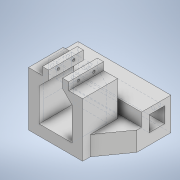
# Autodesk Inventor part: Motorhalterig
Saved by Autodesk Inventor 2021 (Build 250183000, 183)
## iProperties
Created: 2024-01-31
Part Number: Motorhalterig
Material: Generic
Document SubType Name: Modeling
Designer: Lukas
Density: 1 g/cm^3
Appearance: Default
Author: Lukas
Autodesk Inventor part; units mm, degrees
ref_plane "YZ Plane" through (0, 0, 0) normal (1, 0, 0) x (0, 1, 0)
ref_plane "XZ Plane" through (0, 0, 0) normal (0, 1, 0) x (-1, 0, 0)
ref_plane "XY Plane" through (0, 0, 0) normal (0, 0, 1) x (1, 0, 0)
sketch "Sketch1" plane through (0, 0, 0) normal (0, 0, 1) x (1, 0, 0)
  line L0 (-21.25, 21.25) -> (21.25, 21.25)
  line L1 (21.25, 21.25) -> (21.25, -21.25)
  line L2 (21.25, -21.25) -> (-21.25, -21.25)
  line L3 (-21.25, -21.25) -> (-21.25, 21.25)
  line L4 (-35, -35) -> (35, -35)
  line L5 (35, -35) -> (35, 35)
  line L6 (35, 35) -> (-35, 35)
  line L7 (-35, 35) -> (-35, -35)
  line L8 (-9, 35) -> (-9, 21.25)
  line L9 (9, 21.25) -> (9, 35)
  point P0 (0, 0)
  point P1 (-21.25, 0)
  point P2 (0, 21.25)
  point P3 (-35, 0)
  point P4 (0, 35)
  dimension "d0" = 42.5
  dimension "d1" = 9
  dimension "d3" = 70
  dimension "d17" = 18
  constraints: 20 end point, 6 perpendicular, 4 midpoint, 4 parallel, 4 point on line, 2 horizontal, 2 horizontal alignment, 2 vertical alignment
  measures "d0" distance of L0.start L0.end
  measures "d1" distance from line of point (0, 21.25) L8
  measures "d3" distance of L6.end L4.start
  measures "d17" distance between parallel lines of L9 L8
extrude "Extrusion1" add sketch "Sketch1" along normal blind 45 contours L3 L2 L1 L0 L9 L6 L5 L4 L7 L8
sketch "Sketch4" plane through (0, 0, 0) normal (1, 0, 0) x (0, 1, 0)
  line L0 (-0.9, -15.9) -> (-21, -15.9)
  line L1 (-21, -15.9) -> (-21, -36)
  line L2 (-21, -36) -> (-0.9, -36)
  line L3 (-0.9, -36) -> (-0.9, -15.9)
  line L4 (-35, 0) -> (-35, 45) projected
  line L5 (7, -6) -> (7, -44)
  line L6 (7, -44) -> (-35, -44)
  line L7 (-35, -44) -> (-35, 0)
  line L8 (7, -6) -> (-10, -6)
  line L9 (-10, -6) -> (-10, 0)
  line L10 (-10, 0) -> (-35, 0)
  point P0 (0, 0)
  dimension "d18" = 20.1
  dimension "d20" = 14
  dimension "d21" = 42
  dimension "d22" = 38
  dimension "d30" = 8
  dimension "d31" = 6
  dimension "d32" = 25
  constraints: 20 end point, 4 horizontal, 3 parallel, 2 perpendicular, 2 vertical
  measures "d18" distance of L2.end L0.start
  measures "d20" distance between parallel lines of L1 L4
  measures "d21" distance of L5.end L6.end
  measures "d22" distance of L5.start L5.end
  measures "d30" distance between parallel lines of L6 L2
  measures "d31" distance of L8.end L9.end
  measures "d32" distance between parallel lines of L7 L9
extrude "Extrusion5" add sketch "Sketch4" along normal mid plane 120
sketch "Sketch5" plane through (60, 7, -44) normal (0, 0, -1) x (-1, 0, 0)
  circle A0 centre (15, -17.95) radius 2.15
  circle A1 centre (105, -17.95) radius 2.15
  line L0 (120, -7.9) -> (120, -7.9) projected
  line L1 (120, 0) -> (120, -42) projected
  line L2 (0, -42) -> (0, 0) projected
  line L3 (120, -28) -> (120, -7.9) projected
  point P0 (60, -7)
  point P1 (120, -21)
  point P2 (120, -17.95)
  dimension "d27" = 4.3
  dimension "d58" = 15
  dimension "d59" = 15
  constraints: 2 centre point, 2 horizontal alignment, 2 midpoint, 1 equal radius
  measures "d27" diameter of A0
  measures "d58" distance from line of L1 A1.centre
  measures "d59" distance from line of L2 A0.centre
extrude "Extrusion6" cut sketch "Sketch5" against normal blind 18
sketch "Sketch6" plane through (9, 35, 0) normal (0, 1, 0) x (1, 0, 0)
  line L0 (26, 0) -> (0, 0) projected
  line L1 (0, 0) -> (8, 0)
  line L2 (8, 0) -> (8, -45)
  line L3 (8, -45) -> (0, -45)
  line L4 (0, -45) -> (0, 0)
  line L5 (-18, 0) -> (-18, -45) projected
  line L6 (-18, 0) -> (-26, 0)
  line L7 (-26, 0) -> (-26, -45)
  line L8 (-26, -45) -> (-18, -45)
  line L9 (-18, -45) -> (-18, 0)
  line L10 (26, -45) -> (0, -45) projected
  point P0 (-9, 0)
  dimension "d39" = 8
  constraints: 16 end point, 4 parallel, 2 horizontal, 2 perpendicular, 2 point on line, 1 collinear
  measures "d39" distance between parallel lines of L4 L2
extrude "Extrusion7" add sketch "Sketch6" along normal blind 10
sketch "Sketch7" plane through (17, 35, 45) normal (1, 0, 0) x (0, 0, -1)
  circle A0 centre (12.5, 5) radius 1.6
  circle A1 centre (32.5, 5) radius 1.6
  line L0 (45, 10) -> (0, 10) projected
  point P0 (45, -35)
  point P1 (22.5, 10)
  dimension "d42" = 20
  dimension "d43" = 10
  dimension "d44" = 5
  dimension "d45" = 3.2
  constraints: 2 centre point, 1 equal radius, 1 horizontal alignment, 1 midpoint
  measures "d42" distance of A1.centre A0.centre
  measures "d43" horizontal distance of point (22.5, 10) A0.centre
  measures "d44" distance from line of L0 A0.centre
  measures "d45" diameter of A0
extrude "Extrusion8" cut sketch "Sketch7" against normal through all
sketch "Sketch8" plane through (-17, 35, 0) normal (-1, 0, 0) x (0, 0, 1)
  circle A0 centre (12.5, 5) radius 1.6 projected
  circle A1 centre (32.5, 5) radius 1.6 projected
  circle A2 centre (12.5, 5) radius 2.1
  circle A3 centre (32.5, 5) radius 2.1
  point P0 (0, -35)
  dimension "d48" = 4.2
  constraints: 2 centre point, 2 coincident, 1 equal radius
  measures "d48" diameter of A3
extrude "Extrusion9" cut sketch "Sketch8" against normal blind 6
chamfer "Chamfer1" distance 25 angle 45 1 edges at (-35, -22.5, 0)
chamfer "Chamfer2" distance 35 distance2 25 1 edges at (35, -22.5, 0) measured on face at (35, -3.3333, 30)
chamfer "Chamfer3" distance 12.25 angle 45 2 edges at (-9, 21.25, 22.5) (9, 21.25, 22.5)
equation "\"d1\" = 0.5 * d17"
equation "\"d59\" = d58"
equation "\"d43\" = 0.5 * d42"
body "Solid1"
